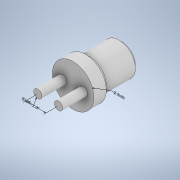
# Autodesk Inventor part: Деталь4
Saved by Autodesk Inventor 2021 (Build 250183000, 183)
## iProperties
Created: 2022-10-18
Part Number: Деталь4
Material: Типовые
Document SubType Name: Modeling
Designer: 22-91-12
Density: 1 g/cm^3
Appearance: По умолчанию
Author: 22-91-12
Autodesk Inventor part; units mm, degrees
ref_plane "YZ Plane" through (0, 0, 0) normal (1, 0, 0) x (0, 1, 0)
ref_plane "XZ Plane" through (0, 0, 0) normal (0, 1, 0) x (-1, 0, 0)
ref_plane "XY Plane" through (0, 0, 0) normal (0, 0, 1) x (1, 0, 0)
sketch "Эскиз1" plane through (0, 0, 0) normal (0, 1, 0) x (-1, 0, 0)
  line L0 (3.1376, 6.642) -> (-6.8624, 6.642)
  line L1 (-6.8624, 6.642) -> (-6.8624, 3.642)
  line L2 (3.1376, 6.642) -> (3.1376, 3.642)
  line L3 (3.1376, 3.642) -> (2.077, 2.5813)
  line L4 (-6.8624, 3.642) -> (-5.8017, 2.5813)
  line L5 (2.077, 2.5813) -> (2.077, -4.4187)
  line L6 (2.077, -4.4187) -> (1.3699, -5.1258)
  line L7 (-5.8017, 2.5813) -> (-5.8017, -4.4187)
  line L8 (-5.8017, -4.4187) -> (-5.0946, -5.1258)
  line L9 (1.3699, -5.1258) -> (-5.0946, -5.1258)
  line L10 (-1.8624, 6.642) -> (-1.8624, -5.1258)
  point P0 (0, 0)
  constraints: 22 end point, 4 vertical, 2 horizontal, 2 midpoint
revolve "Вращение1" add sketch "Эскиз1" angle 360 about axis through (1.8624, 0, 6.642) along (0, 0, -1) contours L2 L3 L5 L6 L9 L10 L0
sketch "Эскиз6" plane through (1.8624, 0, 6.642) normal (0, 0, 1) x (1, 0, 0)
  circle A0 centre (0, 0) radius 3.2322 projected
  circle A1 centre (-2.5, 0) radius 1
  circle A2 centre (2.5, 0) radius 1
  constraints: 2 centre point
sketch3d "3D эскиз3"
  line L0 (-0.6376, 0, 6.642) -> (-0.6376, 0, 12.642)
sweep "Сдвиг2" add profiles "Эскиз6" path "3D эскиз3" contours A0 A2 | A0 A2 | A1 A0 | A0 A1
